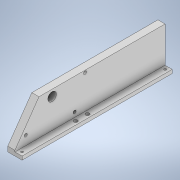
# Autodesk Inventor part: s_base4
Saved by Autodesk Inventor 2022 (Build 260153000, 153)
## iProperties
Created: 2021-08-20
Part Number: s_base4
Material: 一般
Document SubType Name: Modeling
Designer: yuta0
Density: 1 g/cm^3
Appearance: 既定
Author: yuta0
Autodesk Inventor part; units mm, degrees
ref_plane "YZ Plane" through (0, 0, 0) normal (1, 0, 0) x (0, 1, 0)
ref_plane "XZ Plane" through (0, 0, 0) normal (0, 1, 0) x (-1, 0, 0)
ref_plane "XY Plane" through (0, 0, 0) normal (0, 0, 1) x (1, 0, 0)
sketch "スケッチ1" plane through (0, 0, 0) normal (0, 0, 1) x (1, 0, 0)
  line L0 (-20, -2.5) -> (20, -2.5)
  line L1 (20, -2.5) -> (20, 2.5)
  line L2 (-20, 2.5) -> (-20, -2.5)
  line L3 (-20, -2.5) -> (20, 2.5) construction
  line L4 (20, -2.5) -> (-20, 2.5) construction
  line L5 (-10, 2.5) -> (10, 2.5)
  line L6 (10, 2.5) -> (10, 52.5)
  line L7 (10, 52.5) -> (-10, 52.5)
  line L8 (-10, 52.5) -> (-10, 2.5)
  line L9 (-10, 2.5) -> (10, 52.5) construction
  line L10 (10, 2.5) -> (-10, 52.5) construction
  line L11 (20, 2.5) -> (10, 2.5)
  line L12 (-10, 2.5) -> (-20, 2.5)
  line L13 (0, 52.5) -> (0, -2.5)
  point P0 (0, 0)
  point P1 (0, 27.5)
  point P2 (0, 27.5)
  point P3 (0, 0)
  dimension "d0" = 20
  dimension "d1" = 50
  dimension "d2" = 5
  dimension "d3" = 10
  constraints: 28 end point, 8 midpoint, 5 parallel, 2 horizontal, 2 perpendicular, 1 vertical alignment
  measures "d0" distance of L6.end L7.end
  measures "d1" distance of L5.end L6.end
  measures "d2" distance of L0.end L1.end
  measures "d3" distance between parallel lines of L8 L2
extrude "押し出し1" add sketch "スケッチ1" along normal mid plane 210 contours L13 L5 L11 L1 L0 | L13 L7 L6 L5
sketch "スケッチ4" plane through (0, -2.5, 105) normal (-1, 0, 0) x (0, 0, 1)
  line L0 (0, 7) -> (-33.61, 55)
  line L1 (-210, 55) -> (0, 55) projected
  line L2 (0, 55) -> (0, 0) projected
  line L3 (0, 5) -> (-210, 5) projected
  point P0 (-105, 2.5)
  dimension "d18" = 35
  dimension "d21" = 2
  constraints: 2 end point, 2 point on line
  measures "d18" angle of L2 L0
  measures "d21" distance from line of L3 L0.start
extrude "押し出し3" cut sketch "スケッチ4" against normal through all
sketch "スケッチ5" plane through (10, 2.5, -105) normal (1, 0, 0) x (0, 0, -1)
  circle A0 centre (-158, 41) radius 6.05
  line L0 (0, 0) -> (-210, 0) projected
  line L1 (-210, 0) -> (-210, 2) projected
  point P0 (-105, -2.5)
  dimension "d22" = 12.1
  dimension "d23" = 41
  dimension "d37" = 52
  constraints: 1 centre point
  measures "d22" diameter of A0
  measures "d23" distance from line of L0 A0.centre
  measures "d37" distance from line of L1 A0.centre
extrude "押し出し4" cut sketch "スケッチ5" against normal blind 10
sketch "スケッチ6" plane through (10, 2.5, 105) normal (0, 1, 0) x (1, 0, 0)
  line L0 (10, 210) -> (10, 0) projected
  line L1 (10, 0) -> (0, 0) projected
  line L2 (0, 210) -> (10, 210) projected
  point P0 (-10, 105)
  point P1 (5, 205)
  point P2 (5, 5)
  point P3 (5, 79.86)
  point P4 (5, 96.483)
  dimension "d27" = 5
  dimension "d28" = 5
  dimension "d29" = 5
  dimension "d50" = 16.623
  dimension "d51" = 74.86
  constraints: 1 vertical alignment
  measures "d27" distance from line of L0 point (5, 205)
  measures "d28" distance from line of L1 point (5, 5)
  measures "d29" distance from line of L2 point (5, 205)
  measures "d50" distance of point (5, 79.86) point (5, 96.483)
  measures "d51" distance of point (5, 5) point (5, 79.86)
hole "穴2" at (15, 2.5, -100) at (15, 2.5, 100) direction (0, -1, 0) diameter 3.2 end through all clearance for "Socket Head Cap Screw" size "M3" standard "Ansi Metric M Profile"
hole "穴4" at (15, 2.5, 25.14) at (15, 2.5, 8.517) direction (0, -1, 0) diameter 5.2 end through all
sketch "スケッチ8" plane through (10, 2.5, -105) normal (1, 0, 0) x (0, 0, -1)
  circle A0 centre (-158, 41) radius 6.05 projected
  circle A1 centre (-158, 41) radius 46.5
  point P0 (-105, -2.5)
  point P1 (-194.9335, 12.7482)
  point P2 (-126.6367, 6.6693)
  point P3 (-111.8887, 47)
  dimension "d59" = 93
  dimension "d62" = 95
  dimension "d63" = 55
  dimension "d64" = 6
  constraints: 3 point on circle, 1 centre point, 1 coincident
  measures "d59" diameter of A1
  measures "d64" vertical distance of A1.centre point (-111.889, 47)
hole "穴5" at (10, 15.2482, 89.9335) at (10, 9.1693, 21.6367) at (10, 49.5, 6.8887) direction (-1, 0, 0) diameter 4.3 end through all
